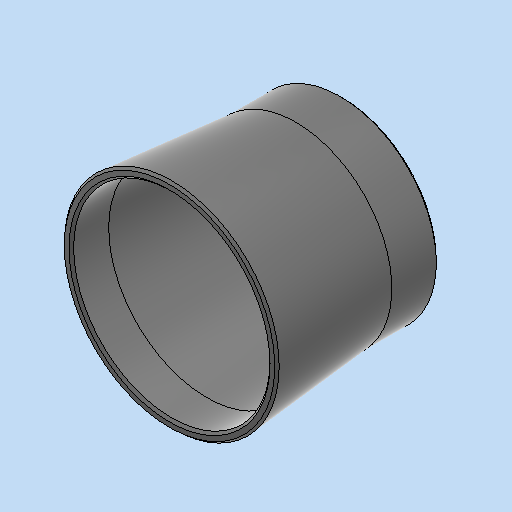
# Autodesk Inventor part: Takumar-to-RisingCam
Saved by Autodesk Inventor 2025 (Build 290162000, 162)
## iProperties
Created: 2025-02-19
Part Number: Takumar-to-RisingCam
Material: ABS Plastic
Document SubType Name: Modeling
Designer: kuzmin
Density: 1.06 g/cm^3
Appearance: Smooth - Black
Author: kuzmin
Autodesk Inventor part; units mm, degrees
ref_plane "YZ Plane" through (0, 0, 0) normal (1, 0, 0) x (0, 1, 0)
ref_plane "XZ Plane" through (0, 0, 0) normal (0, 1, 0) x (-1, 0, 0)
ref_plane "XY Plane" through (0, 0, 0) normal (0, 0, 1) x (1, 0, 0)
sketch "Sketch1" plane through (0, 0, 0) normal (0, 1, 0) x (-1, 0, 0)
  line L0 (0, 0) -> (0, 37)
  line L1 (20.55, 0) -> (20.55, 10)
  line L2 (20.55, 10) -> (23, 37)
  line L3 (23, 37) -> (21, 37)
  line L4 (18.55, 0) -> (20.55, 0)
  line L5 (0, 0) -> (18.55, 0) construction
  line L6 (21, 37) -> (0, 37) construction
  line L7 (21, 37) -> (21, 29)
  line L8 (21, 29) -> (18.55, 0)
  dimension "d0" = 41.1
  dimension "d1" = 42
  dimension "d2" = 37
  dimension "d3" = 10
  dimension "d4" = 8
  dimension "d11" = 2
  dimension "d12" = 2
  constraints: 19 end point, 3 horizontal, 3 vertical, 1 parallel
  measures "d0" diameter of L1.start L0
  measures "d1" diameter of L7 L0
  measures "d2" distance of L0.start L0.end
  measures "d3" distance of L1.start L1.end
  measures "d4" distance of L3.end L7.end
  measures "d11" distance of L4.start L1.start
  measures "d12" distance of L2.end L3.end
revolve "Revolution1" add sketch "Sketch1" angle 360 about axis through (0, 0, 0) along (0, 0, 1)
chamfer "Chamfer1" distance 0.5 angle 45 4 edges at (20.55, 0, 0) (18.55, 0, 0) (23, 0, 37) (21, 0, 37)
body "Solid1"
